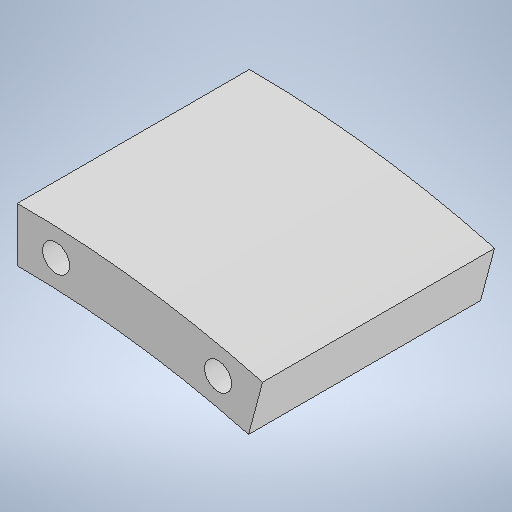
# Autodesk Inventor part: 3D_base-connect
Saved by Autodesk Inventor 2025 (Build 290162000, 162)
## iProperties
Created: 2024-07-27
Part Number: 3D_base-connect
Material: 一般
Document SubType Name: Modeling
Designer: 8326d
Density: 1 g/cm^3
Appearance: 既定
Author: 8326d
Autodesk Inventor part; units mm, degrees
ref_plane "YZ Plane" through (0, 0, 0) normal (1, 0, 0) x (0, 1, 0)
ref_plane "XZ Plane" through (0, 0, 0) normal (0, 1, 0) x (-1, 0, 0)
ref_plane "XY Plane" through (0, 0, 0) normal (0, 0, 1) x (1, 0, 0)
sketch "スケッチ1" plane through (0, 0, 0) normal (0, 0, 1) x (1, 0, 0)
  arc A0 (31.7053, 118.3259) -> (0, 122.5) centre (0, 0) ccw
  line L0 (0, 0) -> (0, 122.5) construction
  line L1 (0, 0) -> (122.5, 0) construction
  line L2 (0, 0) -> (31.7053, 118.3259) construction
  arc A1 (29.8936, 111.5644) -> (0, 115.5) centre (0, 0) ccw
  line L3 (0, 122.5) -> (0, 115.5)
  line L4 (31.7053, 118.3259) -> (29.8936, 111.5644)
  dimension "d0" = 122.5
  dimension "d1" = 90
  dimension "d2" = 15
  dimension "d3" = 7
  constraints: 10 end point, 4 point on circle, 2 centre point, 2 collinear, 2 point on line, 1 coincident, 1 horizontal, 1 perpendicular
  measures "d0" radius of A0
  measures "d1" angle of L1 L0
  measures "d2" angle of L2 L0
  measures "d3" radial gap between concentric circles of A0 A1
extrude "押し出し1" add sketch "スケッチ1" along normal blind 30
sketch "スケッチ2" plane through (0, 0, 30) normal (0, 0, 1) x (1, 0, 0)
  arc A0 (31.7053, 118.3259) -> (0, 122.5) centre (0, 0) ccw projected
  arc A1 (30.7995, 114.9452) -> (0, 119) centre (0, 0) ccw construction
  line L0 (0, 122.5) -> (0, 115.5) projected
  line L1 (29.8936, 111.5644) -> (31.7053, 118.3259) projected
  point P0 (4.9989, 118.895)
  point P1 (25.9437, 116.1375)
  point P2 (0, 119)
  point P3 (30.7995, 114.9452)
  dimension "d6" = 3.5
  dimension "d7" = 5
  dimension "d8" = 5
  constraints: 4 point on circle, 2 midpoint, 1 centre point
  measures "d6" radial gap between concentric circles of A0 A1
  measures "d7" distance of point (0, 119) point (4.999, 118.895)
  measures "d8" distance of point (30.799, 114.945) point (25.944, 116.138)
hole "穴1" at (4.9989, 118.895, 30) at (25.9437, 116.1375, 30) direction (0, 0, -1) diameter 3.5 depth 8 tip angle 118
equation "\"d8\" = d7"
